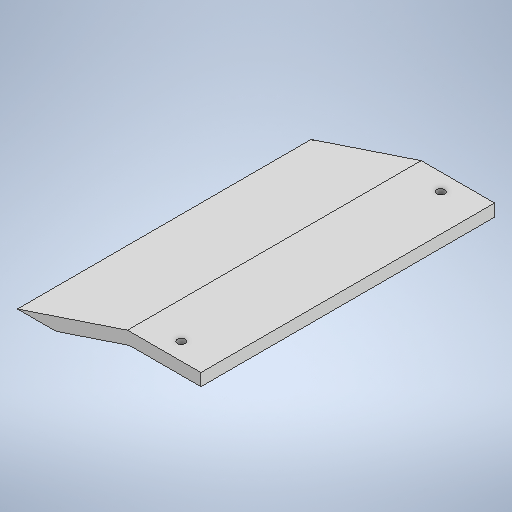
# Autodesk Inventor part: 排出スロープ
Saved by Autodesk Inventor 2026.2 (Build 302298010, 298A)
## iProperties
Created: 2026-05-06
Part Number: 排出スロープ
Material: 一般
Document SubType Name: Modeling
Designer: Yagis
Density: 1 g/cm^3
Appearance: 既定
Author: Yagis
Autodesk Inventor part; units mm, degrees
ref_plane "YZ Plane" through (0, 0, 0) normal (1, 0, 0) x (0, 1, 0)
ref_plane "XZ Plane" through (0, 0, 0) normal (0, 1, 0) x (-1, 0, 0)
ref_plane "XY Plane" through (0, 0, 0) normal (0, 0, 1) x (1, 0, 0)
sketch "スケッチ1" plane through (0, 0, 0) normal (0, 0, 1) x (1, 0, 0)
  line L0 (0, 0) -> (45, 15)
  line L1 (45, 15) -> (75, 15)
  line L2 (75, 15) -> (75, 10)
  line L3 (75, 10) -> (45.8114, 10)
  line L4 (45.8114, 10) -> (15.8114, 0)
  line L5 (15.8114, 0) -> (0, 0)
  dimension "d0" = 15
  dimension "d1" = 5
  dimension "d2" = 5
  dimension "d21" = 30
  dimension "d27" = 30
  constraints: 12 end point, 2 horizontal, 2 perpendicular, 1 parallel
  measures "d0" vertical distance of L0.start L0.end
  measures "d1" distance between parallel lines of L3 L1
  measures "d2" distance between parallel lines of L4 L0
  measures "d21" distance of L0.end L1.end
  measures "d27" horizontal distance of L3.end L4.end
extrude "押し出し1" add sketch "スケッチ1" along normal blind 120
sketch "スケッチ3" plane through (45, 15, 0) normal (0, 1, 0) x (1, 0, 0)
  line L0 (30, 0) -> (30, -120) projected
  line L1 (30, 0) -> (0, 0) projected
  line L2 (30, -120) -> (0, -120) projected
  point P0 (-45, 0)
  point P1 (15, -7)
  point P2 (30, -80)
  point P3 (15, -113)
  point P4 (15, -120)
  dimension "d12" = 15
  dimension "d13" = 7
  dimension "d23" = 106
  constraints: 1 midpoint, 1 vertical alignment
  measures "d12" distance from line of point (15, -7) L0
  measures "d13" distance from line of point (15, -7) L1
  measures "d23" distance of point (15, -113) point (15, -7)
hole "穴1" at (60, 15, 7) at (60, 15, 113) direction (0, -1, 0) diameter 3.2 depth 10 tip angle 118
